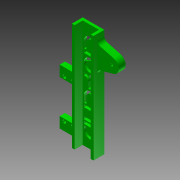
# Autodesk Inventor part: TabletMount-Mast-Right
Saved by Autodesk Inventor 2012 (Build 160160000, 160)
## iProperties
Created: 2013-10-06
Part Number: TabletMount-Mast-Right
Material: Default
Document SubType Name: Modeling
Designer: joe_000
Density: 1 g/cm^3
WallThickness: 0.125 in
HingeAngle: 75.00 deg
HingeLength: 0.750 in
Length: 5.000 in
HingeHoleDiameter: 0.118 in
Author: joe_000
Autodesk Inventor part; units mm, degrees
ref_plane "YZ Plane" through (0, 0, 0) normal (1, 0, 0) x (0, 1, 0)
ref_plane "XZ Plane" through (0, 0, 0) normal (0, 1, 0) x (-1, 0, 0)
ref_plane "XY Plane" through (0, 0, 0) normal (0, 0, 1) x (1, 0, 0)
sketch "Sketch1" plane through (0, 0, 0) normal (0, 1, 0) x (-1, 0, 0)
  line L0 (0, 0) -> (0, 12.7)
  line L1 (0, 12.7) -> (3.175, 12.7)
  line L2 (3.175, 12.7) -> (3.175, 3.175)
  line L3 (3.175, 3.175) -> (22.225, 3.175)
  line L4 (22.225, 3.175) -> (22.225, 12.7)
  line L5 (22.225, 12.7) -> (25.4, 12.7)
  line L6 (25.4, 12.7) -> (25.4, 0)
  line L7 (25.4, 0) -> (0, 0)
  dimension "WallThickness" = 3.175
  dimension "d1" = 19.05
  dimension "d2" = 9.525
  dimension "d3" = 3.175
  dimension "d4" = 3.175
  constraints: 16 end point, 5 parallel, 2 collinear, 1 perpendicular, 1 vertical
  measures "WallThickness" distance of L0.end L1.end
  measures "d1" distance of L2.end L3.end
  measures "d2" distance of L1.end L2.end
  measures "d3" distance between parallel lines of L7 L3
  measures "d4" distance between parallel lines of L6 L4
extrude "Extrusion1" add sketch "Sketch1" along normal blind 127
sketch "Sketch2" plane through (0, 0, 0) normal (0, 0, -1) x (-1, 0, 0)
  line L0 (0, 0) -> (0, 127) projected
  line L1 (0, 116.8008) -> (-19.05, 111.6964)
  line L2 (0, 90.5114) -> (-19.05, 95.6158)
  arc A0 (-19.05, 111.6964) -> (-19.05, 95.6158) centre (-16.8956, 103.6561) ccw
  dimension "HingeAngle" = 75
  dimension "d8" = 75
  dimension "HingeLength" = 19.05
  dimension "d10" = 19.05
  constraints: 4 end point, 2 point on circle, 2 point on line, 1 centre point, 1 tangent
  measures "HingeAngle" angle of L0 L2
  measures "d8" angle of L0 L1
  measures "HingeLength" distance from line of L0 L2.end
  measures "d10" horizontal distance of L1.start L1.end
extrude "Extrusion2" add sketch "Sketch2" against normal blind 8.2127
hole "Hole1" at (16.8956, 103.6561, 0) direction (0, 0, 1) diameter 3 end through all
sketch "Sketch3" plane through (0, 0, 0) normal (0, 0, -1) x (-1, 0, 0)
  line L0 (25.4, 0) -> (0, 0) projected
  line L1 (25.4, 0) -> (25.4, 127) projected
  line L2 (25.4, 71.5612) -> (46.2, 71.5612)
  line L3 (46.2, 71.5612) -> (46.2, 58.8612)
  line L4 (46.2, 58.8612) -> (25.4, 58.8612)
  line L5 (25.4, 58.8612) -> (25.4, 71.5612)
  line L6 (25.4, 19.05) -> (46.2, 19.05)
  line L7 (46.2, 19.05) -> (46.2, 6.35)
  line L8 (46.2, 6.35) -> (25.4, 6.35)
  line L9 (25.4, 6.35) -> (25.4, 19.05)
  line L10 (35.8, 71.5612) -> (35.8, 58.8612)
  point P0 (30.8, 61.8612)
  dimension "d21" = 20.8
  dimension "d22" = 12.7
  dimension "d23" = 39.8112
  dimension "d24" = 6.35
  dimension "d25" = 5
  dimension "d26" = 3
  constraints: 18 end point, 4 parallel, 2 collinear, 2 horizontal, 2 midpoint, 2 perpendicular, 2 point on line
  measures "d21" distance of L2.start L2.end
  measures "d22" distance of L2.end L3.end
  measures "d23" distance between parallel lines of L6 L4
  measures "d24" distance between parallel lines of L0 L8
  measures "d25" distance from line of point (30.8, 61.861) L10
  measures "d26" distance from line of point (30.8, 61.861) L4
extrude "Extrusion3" add sketch "Sketch3" against normal blind 6.35
fillet "Fillet1" radius 5.08 4 edges at (-25.4, 71.5612, 3.175) (-25.4, 65.2112, 6.35) (-25.4, 12.7, 6.35) (-25.4, 6.35, 3.175)
hole "Hole2" at (-30.8, 61.8612, 0) direction (0, 0, 1) diameter 4 end through all
pattern_linear "Rectangular Pattern1" count 2 spacing 10 along (-1, 0, 0) count 2 spacing 45.8 along (0, -1, 0) of "Hole2"
fillet "Fillet2" radius 5.08 2 edges at (0, 116.8008, 4.1063) (0, 90.5114, 4.1063)
sketch "Sketch5" plane through (0, 0, 0) normal (0, 0, -1) x (-1, 0, 0)
  line L0 (5.5358, 9.9994) -> (5.5358, 143.0184) construction
  line L1 (5.5358, 143.0184) -> (24.6134, 143.0184) construction
  line L2 (24.6134, 143.0184) -> (24.6134, 9.9994) construction
  line L3 (24.6134, 9.9994) -> (5.5358, 9.9994) construction
  line L4 (5.5358, 18.2981) -> (5.5358, 25.3498)
  line L5 (5.5358, 25.3498) -> (20.7979, 25.3498)
  line L6 (20.7979, 25.3498) -> (20.7979, 22.2929)
  line L7 (20.7979, 22.2929) -> (8.5043, 22.2929)
  line L8 (8.5043, 22.2929) -> (8.5154, 19.5561)
  line L9 (8.5154, 19.5561) -> (8.5154, 18.9051)
  spline S0 degree 2 poles (8.5154, 18.9051) (8.5154, 16.6207) (8.703, 16.3669) knots 0 0 0 1 1 1
  spline S1 degree 2 poles (8.703, 16.3669) (9.0782, 14.9985) (10.281, 14.0494) knots 0 0 0 1 1 1
  spline S2 degree 2 poles (10.281, 14.0494) (11.7377, 13.0342) (13.1723, 13.0342) knots 0 0 0 1 1 1
  spline S3 degree 2 poles (13.1723, 13.0342) (14.9601, 13.0342) (16.4499, 14.4136) knots 0 0 0 1 1 1
  spline S4 degree 2 poles (16.4499, 14.4136) (17.3217, 15.3406) (17.5093, 16.0027) knots 0 0 0 1 1 1
  spline S5 degree 2 poles (17.5093, 16.0027) (17.8403, 16.6649) (17.8403, 18.2981) knots 0 0 0 1 1 1
  line L10 (17.8403, 18.2981) -> (17.8403, 20.428)
  line L11 (17.8403, 20.428) -> (20.7979, 20.428)
  line L12 (20.7979, 20.428) -> (20.7979, 17.8788)
  spline S6 degree 2 poles (20.7979, 17.8788) (20.7979, 15.0426) (19.3081, 13.0783) knots 0 0 0 1 1 1
  spline S7 degree 2 poles (19.3081, 13.0783) (18.1824, 11.6658) (17.2775, 11.1802) knots 0 0 0 1 1 1
  spline S8 degree 2 poles (17.2775, 11.1802) (15.3905, 9.9994) (13.4151, 9.9994) knots 0 0 0 1 1 1
  line L13 (13.4151, 9.9994) -> (12.9737, 9.9994)
  spline S9 degree 2 poles (12.9737, 9.9994) (10.2259, 9.9994) (7.9195, 12.0631) knots 0 0 0 1 1 1
  spline S10 degree 2 poles (7.9195, 12.0631) (6.7055, 13.3101) (6.3855, 14.1046) knots 0 0 0 1 1 1
  spline S11 degree 2 poles (6.3855, 14.1046) (6.0765, 14.6785) (5.7896, 15.6827) knots 0 0 0 1 1 1
  spline S12 degree 2 poles (5.7896, 15.6827) (5.5358, 16.5876) (5.5358, 18.2981) knots 0 0 0 1 1 1
  spline S13 degree 2 poles (5.5579, 34.6306) (5.5579, 38.2944) (8.5816, 40.7663) knots 0 0 0 1 1 1
  spline S14 degree 2 poles (8.5816, 40.7663) (9.1996, 41.2188) (9.63, 41.4285) knots 0 0 0 1 1 1
  spline S15 degree 2 poles (9.63, 41.4285) (10.1486, 41.7154) (11.0315, 41.9802) knots 0 0 0 1 1 1
  spline S16 degree 2 poles (11.0315, 41.9802) (12.0909, 42.3003) (13.9117, 42.3003) knots 0 0 0 1 1 1
  line L14 (13.9117, 42.3003) -> (20.7979, 42.3003)
  line L15 (20.7979, 42.3003) -> (20.7979, 39.2434)
  line L16 (20.7979, 39.2434) -> (13.5807, 39.2434)
  spline S17 degree 2 poles (13.5807, 39.2434) (9.9389, 39.2434) (8.703, 35.9549) knots 0 0 0 1 1 1
  spline S18 degree 2 poles (8.703, 35.9549) (8.4933, 35.1934) (8.4823, 34.6306) knots 0 0 0 1 1 1
  spline S19 degree 2 poles (8.4823, 34.6306) (8.4933, 34.0568) (8.703, 33.3174) knots 0 0 0 1 1 1
  spline S20 degree 2 poles (8.703, 33.3174) (9.9389, 30.0178) (13.5807, 30.0178) knots 0 0 0 1 1 1
  line L17 (13.5807, 30.0178) -> (20.7979, 30.0178)
  line L18 (20.7979, 30.0178) -> (20.7979, 26.9499)
  line L19 (20.7979, 26.9499) -> (13.9117, 26.9499)
  spline S21 degree 2 poles (13.9117, 26.9499) (12.0909, 26.9499) (11.0315, 27.2699) knots 0 0 0 1 1 1
  spline S22 degree 2 poles (11.0315, 27.2699) (10.1486, 27.5348) (9.63, 27.8328) knots 0 0 0 1 1 1
  spline S23 degree 2 poles (9.63, 27.8328) (9.1885, 28.0314) (8.5816, 28.4949) knots 0 0 0 1 1 1
  spline S24 degree 2 poles (8.5816, 28.4949) (5.5579, 30.9668) (5.5579, 34.6306) knots 0 0 0 1 1 1
  spline S25 degree 2 poles (5.5468, 49.363) (5.5468, 52.4419) (5.6792, 52.9054) knots 0 0 0 1 1 1
  spline S26 degree 2 poles (5.6792, 52.9054) (5.8227, 54.1524) (6.7276, 55.7194) knots 0 0 0 1 1 1
  spline S27 degree 2 poles (6.7276, 55.7194) (7.2573, 56.5692) (8.3498, 57.5403) knots 0 0 0 1 1 1
  spline S28 degree 2 poles (8.3498, 57.5403) (10.4797, 59.2508) (13.1834, 59.2508) knots 0 0 0 1 1 1
  spline S29 degree 2 poles (13.1834, 59.2508) (14.7725, 59.2508) (16.185, 58.6438) knots 0 0 0 1 1 1
  spline S30 degree 2 poles (16.185, 58.6438) (18.9218, 57.4299) (20.1468, 54.6711) knots 0 0 0 1 1 1
  spline S31 degree 2 poles (20.1468, 54.6711) (20.7979, 53.3909) (20.7979, 50.7314) knots 0 0 0 1 1 1
  line L20 (20.7979, 50.7314) -> (20.7979, 44.2425)
  line L21 (20.7979, 44.2425) -> (20.7316, 43.9004)
  line L22 (20.7316, 43.9004) -> (17.8403, 43.9004)
  line L23 (17.8403, 43.9004) -> (17.8403, 51.0624)
  spline S32 degree 2 poles (17.8403, 51.0624) (17.8403, 52.1991) (17.6307, 52.8281) knots 0 0 0 1 1 1
  spline S33 degree 2 poles (17.6307, 52.8281) (17.0679, 54.4834) (15.9643, 55.267) knots 0 0 0 1 1 1
  spline S34 degree 2 poles (15.9643, 55.267) (14.5518, 56.205) (13.2165, 56.205) knots 0 0 0 1 1 1
  spline S35 degree 2 poles (13.2165, 56.205) (11.8702, 56.205) (10.568, 55.3884) knots 0 0 0 1 1 1
  spline S36 degree 2 poles (10.568, 55.3884) (9.8176, 54.8807) (9.4313, 54.2627) knots 0 0 0 1 1 1
  spline S37 degree 2 poles (9.4313, 54.2627) (8.5043, 53.1482) (8.5043, 51.0624) knots 0 0 0 1 1 1
  line L24 (8.5043, 51.0624) -> (8.5043, 43.9004)
  line L25 (8.5043, 43.9004) -> (5.5468, 43.9004)
  line L26 (5.5468, 43.9004) -> (5.5468, 49.363)
  line L27 (5.5468, 60.8509) -> (5.5468, 70.6504)
  spline S38 degree 2 poles (5.5468, 70.6504) (5.5468, 73.2548) (7.1028, 74.7225) knots 0 0 0 1 1 1
  spline S39 degree 2 poles (7.1028, 74.7225) (7.7098, 75.3736) (8.2836, 75.6274) knots 0 0 0 1 1 1
  spline S40 degree 2 poles (8.2836, 75.6274) (9.4313, 76.2013) (10.5238, 76.2013) knots 0 0 0 1 1 1
  line L28 (10.5238, 76.2013) -> (10.9542, 76.2013)
  spline S41 degree 2 poles (10.9542, 76.2013) (12.6206, 76.2013) (14.2207, 74.7556) knots 0 0 0 1 1 1
  spline S42 degree 2 poles (14.2207, 74.7556) (15.1146, 73.8176) (15.3684, 73.0562) knots 0 0 0 1 1 1
  spline S43 degree 2 poles (15.3684, 73.0562) (17.421, 74.9874) (20.7979, 74.9874) knots 0 0 0 1 1 1
  line L29 (20.7979, 74.9874) -> (20.7979, 71.9085)
  line L30 (20.7979, 71.9085) -> (20.5661, 71.9085)
  spline S44 degree 2 poles (20.5661, 71.9085) (18.0721, 71.9085) (16.5933, 69.8779) knots 0 0 0 1 1 1
  spline S45 degree 2 poles (16.5933, 69.8779) (15.7767, 68.7303) (15.7767, 66.8653) knots 0 0 0 1 1 1
  line L31 (15.7767, 66.8653) -> (15.7767, 60.8509)
  line L32 (15.7767, 60.8509) -> (12.8413, 60.8509)
  line L33 (12.8413, 60.8509) -> (12.8413, 70.8491)
  spline S46 degree 2 poles (12.8413, 70.8491) (12.8413, 72.4823) (11.2191, 73.0672) knots 0 0 0 1 1 1
  spline S47 degree 2 poles (11.2191, 73.0672) (10.888, 73.1334) (10.6673, 73.1555) knots 0 0 0 1 1 1
  spline S48 degree 2 poles (10.6673, 73.1555) (9.7624, 73.1555) (9.034, 72.4051) knots 0 0 0 1 1 1
  spline S49 degree 2 poles (9.034, 72.4051) (8.5264, 71.754) (8.5264, 71.0256) knots 0 0 0 1 1 1
  spline S50 degree 2 poles (8.5264, 71.0256) (8.4823, 71.0256) (8.4823, 70.5842) knots 0 0 0 1 1 1
  line L34 (8.4823, 70.5842) -> (8.4823, 60.8509)
  line L35 (8.4823, 60.8509) -> (5.5468, 60.8509)
  line L36 (5.5579, 85.438) -> (5.5579, 85.5373)
  spline S51 degree 2 poles (5.5579, 85.5373) (5.5579, 89.0576) (8.4381, 91.5406) knots 0 0 0 1 1 1
  spline S52 degree 2 poles (8.4381, 91.5406) (10.59, 93.1518) (13.1392, 93.1518) knots 0 0 0 1 1 1
  line L37 (13.1392, 93.1518) -> (13.2386, 93.1518)
  spline S53 degree 2 poles (13.2386, 93.1518) (16.7589, 93.1518) (19.2087, 90.2163) knots 0 0 0 1 1 1
  spline S54 degree 2 poles (19.2087, 90.2163) (20.7979, 88.0755) (20.7979, 85.5152) knots 0 0 0 1 1 1
  line L38 (20.7979, 85.5152) -> (20.7979, 85.4159)
  spline S55 degree 2 poles (20.7979, 85.4159) (20.7979, 81.9177) (17.9397, 79.4347) knots 0 0 0 1 1 1
  spline S56 degree 2 poles (17.9397, 79.4347) (16.7258, 78.5629) (15.7105, 78.2097) knots 0 0 0 1 1 1
  spline S57 degree 2 poles (15.7105, 78.2097) (14.4414, 77.8014) (13.2165, 77.8014) knots 0 0 0 1 1 1
  line L39 (13.2165, 77.8014) -> (13.1172, 77.8014)
  spline S58 degree 2 poles (13.1172, 77.8014) (9.6631, 77.8014) (7.2021, 80.6486) knots 0 0 0 1 1 1
  spline S59 degree 2 poles (7.2021, 80.6486) (5.8227, 82.5798) (5.6572, 84.1689) knots 0 0 0 1 1 1
  spline S60 degree 2 poles (5.6572, 84.1689) (5.5579, 84.6545) (5.5579, 85.438) knots 0 0 0 1 1 1
  spline S61 degree 2 poles (13.1503, 80.8472) (15.1477, 80.8472) (16.6485, 82.4032) knots 0 0 0 1 1 1
  spline S62 degree 2 poles (16.6485, 82.4032) (17.8403, 83.7937) (17.8403, 85.3166) knots 0 0 0 1 1 1
  line L40 (17.8403, 85.3166) -> (17.8403, 85.6145)
  spline S63 degree 2 poles (17.8403, 85.6145) (17.8403, 86.8395) (17.0017, 88.1196) knots 0 0 0 1 1 1
  spline S64 degree 2 poles (17.0017, 88.1196) (16.0305, 89.4328) (14.5407, 89.8963) knots 0 0 0 1 1 1
  spline S65 degree 2 poles (14.5407, 89.8963) (14.1545, 90.0398) (13.1944, 90.106) knots 0 0 0 1 1 1
  spline S66 degree 2 poles (13.1944, 90.106) (11.2522, 90.106) (9.7513, 88.5941) knots 0 0 0 1 1 1
  spline S67 degree 2 poles (9.7513, 88.5941) (8.4933, 87.1705) (8.4933, 85.4821) knots 0 0 0 1 1 1
  spline S68 degree 2 poles (8.4933, 85.4821) (8.4933, 83.4957) (10.1486, 81.9618) knots 0 0 0 1 1 1
  spline S69 degree 2 poles (10.1486, 81.9618) (10.9984, 81.3217) (11.5832, 81.1452) knots 0 0 0 1 1 1
  spline S70 degree 2 poles (11.5832, 81.1452) (12.4109, 80.8472) (13.1503, 80.8472) knots 0 0 0 1 1 1
  line L41 (5.5579, 94.7519) -> (5.5579, 97.8087)
  line L42 (5.5579, 97.8087) -> (20.7979, 97.8087)
  line L43 (20.7979, 97.8087) -> (20.7979, 94.7519)
  line L44 (20.7979, 94.7519) -> (5.5579, 94.7519)
  spline S71 degree 2 poles (5.5468, 104.9266) (5.5468, 108.0055) (5.6792, 108.469) knots 0 0 0 1 1 1
  spline S72 degree 2 poles (5.6792, 108.469) (5.8227, 109.716) (6.7276, 111.2831) knots 0 0 0 1 1 1
  spline S73 degree 2 poles (6.7276, 111.2831) (7.2573, 112.1328) (8.3498, 113.1039) knots 0 0 0 1 1 1
  spline S74 degree 2 poles (8.3498, 113.1039) (10.4797, 114.8144) (13.1834, 114.8144) knots 0 0 0 1 1 1
  spline S75 degree 2 poles (13.1834, 114.8144) (14.7725, 114.8144) (16.185, 114.2075) knots 0 0 0 1 1 1
  spline S76 degree 2 poles (16.185, 114.2075) (18.9218, 112.9936) (20.1468, 110.2347) knots 0 0 0 1 1 1
  spline S77 degree 2 poles (20.1468, 110.2347) (20.7979, 108.9546) (20.7979, 106.295) knots 0 0 0 1 1 1
  line L45 (20.7979, 106.295) -> (20.7979, 99.8062)
  line L46 (20.7979, 99.8062) -> (20.7316, 99.4641)
  line L47 (20.7316, 99.4641) -> (17.8403, 99.4641)
  line L48 (17.8403, 99.4641) -> (17.8403, 106.6261)
  spline S78 degree 2 poles (17.8403, 106.6261) (17.8403, 107.7628) (17.6307, 108.3918) knots 0 0 0 1 1 1
  spline S79 degree 2 poles (17.6307, 108.3918) (17.0679, 110.0471) (15.9643, 110.8306) knots 0 0 0 1 1 1
  spline S80 degree 2 poles (15.9643, 110.8306) (14.5518, 111.7686) (13.2165, 111.7686) knots 0 0 0 1 1 1
  spline S81 degree 2 poles (13.2165, 111.7686) (11.8702, 111.7686) (10.568, 110.952) knots 0 0 0 1 1 1
  spline S82 degree 2 poles (10.568, 110.952) (9.8176, 110.4444) (9.4313, 109.8264) knots 0 0 0 1 1 1
  spline S83 degree 2 poles (9.4313, 109.8264) (8.5043, 108.7118) (8.5043, 106.6261) knots 0 0 0 1 1 1
  line L49 (8.5043, 106.6261) -> (8.5043, 99.4641)
  line L50 (8.5043, 99.4641) -> (5.5468, 99.4641)
  line L51 (5.5468, 99.4641) -> (5.5468, 104.9266)
  constraints: 2 other
extrude "Extrusion4" cut sketch "Sketch5" against normal up to next
sketch "Sketch8" plane through (0, 0, 0) normal (0, 0, -1) x (-1, 0, 0)
  line L0 (4.7839, 86.2929) -> (21.7112, 86.2929)
  line L1 (21.7112, 86.2929) -> (21.7112, 85.0229)
  line L2 (21.7112, 85.0229) -> (4.7839, 85.0229)
  line L3 (4.7839, 85.0229) -> (4.7839, 86.2929)
  dimension "d48" = 1.27
  constraints: 8 end point, 2 parallel, 1 horizontal, 1 perpendicular
  measures "d48" distance of L2.end L0.start
extrude "Extrusion6" add sketch "Sketch8" against normal blind 1.27
equation "\"d1\" = MastWidth"
equation "\"d2\" = 0.5 * MastWidth"
equation "\"d3\" = WallThickness"
equation "\"d4\" = WallThickness"
equation "\"d8\" = HingeAngle"
equation "\"d10\" = HingeLength"
equation "\"d21\" = ServoWidth + ServoTolerance"
equation "\"d23\" = ServoLength + ServoTolerance"
equation "\"d25\" = 0.5 * ServoScrewSpacing"
equation "\"d26\" = ServoScrewOffsetFromSide - 0.5 * ServoTolerance"
equation "\"d39\" = ServoScrewSpacing"
equation "\"d42\" = ServoScrewSpacingLength"
equation "\"d44\" = 0.333333 * MastWidth"
equation "\"ServoTolerance\" = 1"
equation "\"MastWidth\" = 19.05"
equation "\"ServoWidth\" = 19.8"
equation "\"ServoLength\" = 38.8112"
equation "\"ServoScrewSpacing\" = 10"
equation "\"ServoScrewSpacingLength\" = 45.8"
equation "\"ServoScrewOffsetFromSide\" = 3.5"
body "Solid1"
